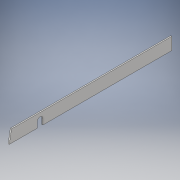
# Autodesk Inventor part: wall-inner-plunger
Saved by Autodesk Inventor 2017 (Build 210142000, 142)
## iProperties
Created: 2017-02-21
Part Number: wall-inner-plunger
Material: Generic
Document SubType Name: Modeling
Designer: John
Density: 1 g/cm^3
Appearance: Default
Author: John
Autodesk Inventor part; units mm, degrees
ref_plane "YZ Plane" through (0, 0, 0) normal (1, 0, 0) x (0, 1, 0)
ref_plane "XZ Plane" through (0, 0, 0) normal (0, 1, 0) x (-1, 0, 0)
ref_plane "XY Plane" through (0, 0, 0) normal (0, 0, 1) x (1, 0, 0)
sketch "Sketch2" plane through (0, 0, 0) normal (0, 1, 0) x (-1, 0, 0)
  line L0 (-1.5, -198.6195) -> (1.5, -198.6195)
  line L1 (1.5, -198.6195) -> (1.5, 198.6195)
  line L2 (1.5, 198.6195) -> (-1.5, 198.6195)
  line L3 (-1.5, 198.6195) -> (-1.5, -198.6195)
  line L4 (-1.5, -198.6195) -> (1.5, 198.6195) construction
  line L5 (1.5, -198.6195) -> (-1.5, 198.6195) construction
  point P0 (0, 0)
  dimension "d0" = 3
  dimension "d1" = 397.239
  constraints: 12 end point, 2 midpoint, 2 parallel, 1 horizontal, 1 perpendicular
  measures "d0" distance of L2.end L1.end
  measures "d1" distance of L1.end L0.end
extrude "Extrusion1" add sketch "Sketch2" along normal blind 30
sketch "Sketch3" plane through (1.5, 0, 198.6195) normal (1, 0, 0) x (0, 0, -1)
  line L0 (397.239, 0) -> (0, 0) projected
  line L1 (68, 0) -> (82, 0)
  line L2 (82, 0) -> (82, 14)
  line L3 (68, 14) -> (68, 0)
  arc A0 (82, 14) -> (68, 14) centre (75, 14) ccw
  arc A1 (68, 14) -> (82, 14) centre (75, 14) ccw construction
  line L4 (0, 0) -> (0, 30) projected
  point P0 (198.6195, 0)
  dimension "d4" = 14
  dimension "d5" = 14
  dimension "d6" = 14
  dimension "d9" = 75
  constraints: 6 end point, 4 point on circle, 2 centre point, 1 horizontal, 1 parallel, 1 perpendicular, 1 point on line
  measures "d4" distance of L3.start L2.end
  measures "d5" distance of L2.end L1.end
  measures "d6" diameter of A0
  measures "d9" distance from line of A0.centre L4
extrude "Extrusion2" cut sketch "Sketch3" against normal through all
sketch "Sketch4" plane through (1.5, 0, -198.6195) normal (1, 0, 0) x (0, 0, -1)
  line L0 (-329.239, 0) -> (-397.239, 0) projected
  line L1 (-397.239, 0) -> (-397.239, 30) projected
  line L2 (-397.239, 0) -> (-397.239, 30)
  line L3 (-397.239, 30) -> (-391.9492, 30)
  line L4 (-397.239, 30) -> (0, 30) projected
  line L5 (-397.239, 0) -> (-391.9492, 30)
  point P0 (-198.6195, 0)
  dimension "d10" = 10
  constraints: 6 end point, 1 point on line, 1 vertical
  measures "d10" angle of L1 L5
extrude "Extrusion3" cut sketch "Sketch4" against normal through all
body "Solid1"
